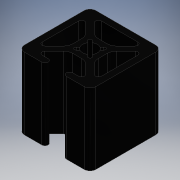
# Autodesk Inventor part: 1001-S-BLACK-FB
Saved by Autodesk Inventor 2017 SP1 (Build 210196100, 196)
## iProperties
Created: 2016-09-13
Part Number: 1001-S-BLACK-FB
Material: 6105-T5
Description: 40 S SHORT SINGLE UNIBEARING ASSEMBLY ON 40-4040 X 75mm
Document SubType Name: Modeling
Designer: BRALEF
Density: 1 g/cm^3
Appearance: BLACK ANODIZED
MATERIAL: 6061-T6
PART PRICE: 44.65
Author: BRALEF
Autodesk Inventor part; units mm, degrees
ref_plane "YZ Plane" through (0, 0, 0) normal (1, 0, 0) x (0, 1, 0)
ref_plane "XZ Plane" through (0, 0, 0) normal (0, 1, 0) x (-1, 0, 0)
ref_plane "XY Plane" through (0, 0, 0) normal (0, 0, 1) x (1, 0, 0)
sketch "Sketch1" plane through (0, 0, 0) normal (0, 1, 0) x (-1, 0, 0)
  arc A0 (4.5172, -1.6395) -> (5.4471, -3.8845) centre (7.6922, -1.6395) ccw
  line L0 (8.7558, -7.1932) -> (5.4471, -3.8845)
  arc A1 (8.7558, -7.1932) -> (10.4902, -6.4748) centre (9.4742, -6.4748) ccw
  line L1 (10.4902, 6.4748) -> (10.4902, -6.4748)
  arc A2 (10.4902, 6.4748) -> (8.7558, 7.1932) centre (9.4742, 6.4748) ccw
  line L2 (5.4471, 3.8845) -> (8.7558, 7.1932)
  arc A3 (5.4471, 3.8845) -> (4.5172, 1.6395) centre (7.6922, 1.6395) ccw
  line L3 (4.5172, -1.6395) -> (4.5172, 1.6395)
  arc A4 (6.4748, -10.4902) -> (7.1932, -8.7558) centre (6.4748, -9.4742) ccw
  line L4 (3.8845, -5.4471) -> (7.1932, -8.7558)
  arc A5 (3.8845, -5.4471) -> (1.6394, -4.5172) centre (1.6394, -7.6922) ccw
  line L5 (-1.6395, -4.5172) -> (1.6394, -4.5172)
  arc A6 (-1.6395, -4.5172) -> (-3.8846, -5.4471) centre (-1.6395, -7.6922) ccw
  line L6 (-7.1932, -8.7558) -> (-3.8846, -5.4471)
  arc A7 (-7.1932, -8.7558) -> (-6.4748, -10.4902) centre (-6.4748, -9.4742) ccw
  line L7 (6.4748, -10.4902) -> (-6.4748, -10.4902)
  arc A8 (-10.4902, -6.4749) -> (-8.7557, -7.1933) centre (-9.4742, -6.4749) ccw
  line L8 (-5.4471, -3.8846) -> (-8.7557, -7.1933)
  arc A9 (-5.4471, -3.8846) -> (-4.5171, -1.6396) centre (-7.6921, -1.6396) ccw
  line L9 (-4.5171, 1.6394) -> (-4.5171, -1.6396)
  arc A10 (-4.5171, 1.6394) -> (-5.4471, 3.8844) centre (-7.6921, 1.6394) ccw
  line L10 (-8.7557, 7.1931) -> (-5.4471, 3.8844)
  arc A11 (-8.7557, 7.1931) -> (-10.4902, 6.4747) centre (-9.4742, 6.4747) ccw
  line L11 (-10.4902, -6.4749) -> (-10.4902, 6.4747)
  arc A12 (1.3405, 2.2319) -> (-1.3405, 2.2319) centre (0, 0) ccw
  line L12 (-1.9692, 2.8605) -> (-1.3405, 2.2319)
  arc A13 (-1.9692, 2.8605) -> (-2.8605, 1.9692) centre (-2.4696, 2.4696) ccw
  line L13 (-2.2319, 1.3405) -> (-2.8605, 1.9692)
  arc A14 (-2.2319, 1.3405) -> (-2.2319, -1.3405) centre (0, 0) ccw
  line L14 (-2.8605, -1.9692) -> (-2.2319, -1.3405)
  arc A15 (-2.8605, -1.9692) -> (-1.9692, -2.8605) centre (-2.4696, -2.4696) ccw
  line L15 (-1.3405, -2.2319) -> (-1.9692, -2.8605)
  arc A16 (-1.3405, -2.2319) -> (1.3405, -2.2319) centre (0, 0) ccw
  line L16 (1.9692, -2.8605) -> (1.3405, -2.2319)
  arc A17 (1.9692, -2.8605) -> (2.8605, -1.9692) centre (2.4696, -2.4696) ccw
  line L17 (2.2319, -1.3405) -> (2.8605, -1.9692)
  arc A18 (2.2319, -1.3405) -> (2.2319, 1.3405) centre (0, 0) ccw
  line L18 (2.8605, 1.9692) -> (2.2319, 1.3405)
  arc A19 (2.8605, 1.9692) -> (1.9692, 2.8605) centre (2.4696, 2.4696) ccw
  line L19 (1.3405, 2.2319) -> (1.9692, 2.8605)
  arc A20 (-4.3561, 10.4904) -> (-4.3452, 12.7001) centre (-4.3451, 11.5952) ccw
  line L20 (-4.3561, 10.4904) -> (-6.4749, 10.4903)
  arc A21 (-6.4749, 10.4903) -> (-7.1933, 8.7559) centre (-6.4749, 9.4743) ccw
  line L21 (-7.1933, 8.7559) -> (-3.8846, 5.4472)
  arc A22 (-3.8846, 5.4472) -> (-1.6396, 4.5173) centre (-1.6396, 7.6923) ccw
  line L22 (-1.6396, 4.5173) -> (1.6397, 4.5173)
  arc A23 (1.6397, 4.5173) -> (3.8848, 5.4472) centre (1.6397, 7.6923) ccw
  line L23 (3.8848, 5.4472) -> (7.1935, 8.7559)
  arc A24 (7.1935, 8.7559) -> (6.475, 10.4903) centre (6.475, 9.4743) ccw
  line L24 (6.475, 10.4903) -> (4.3616, 10.4903)
  arc A25 (4.3616, 12.7001) -> (4.3616, 10.4903) centre (4.3616, 11.5952) ccw
  line L25 (4.3616, 12.7001) -> (10.5011, 12.7001)
  arc A26 (12.7109, 10.4903) -> (10.5011, 12.7001) centre (10.5011, 10.4903) ccw
  line L26 (12.7109, 10.4903) -> (12.7109, -10.5917)
  arc A27 (10.6027, -12.6999) -> (12.7109, -10.5917) centre (10.6027, -10.5917) ccw
  line L27 (10.6027, -12.6999) -> (-10.5992, -12.6999)
  arc A28 (-12.7074, -10.5917) -> (-10.5992, -12.6999) centre (-10.5992, -10.5917) ccw
  line L28 (-12.7074, -10.5917) -> (-12.7074, 10.5919)
  arc A29 (-10.5809, 12.7) -> (-12.7074, 10.5919) centre (-10.5992, 10.5919) ccw
  line L29 (-10.5809, 12.7) -> (-4.3452, 12.7001)
  point P0 (0, 0)
  dimension "d100" = 8.1828
  dimension "d103" = 25.4
  constraints: 60 end point, 60 point on circle, 44 tangent, 30 centre point, 19 equal radius, 16 parallel, 1 horizontal, 1 perpendicular, 1 vertical
  measures "d100" distance between parallel lines of L25 L22
  measures "d103" distance between parallel lines of L27 L25
extrude "Extrusion1" add sketch "Sketch1" along normal mid plane 25.4
body "Solid1"
